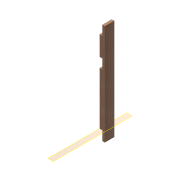
# Autodesk Inventor part: horizontalUnderSink
Saved by Autodesk Inventor 2018 (Build 220112000, 112)
## iProperties
Created: 2018-01-02
Part Number: horizontalUnderSink
Material: Wood (Birch)
Document SubType Name: Modeling
Designer: sawaiz
Density: 0.55 g/cm^3
Appearance: Birch - Natural Polished
Author: sawaiz
Autodesk Inventor part; units mm, degrees
ref_plane "Work Plane1" through (0, 0, 0) normal (0, 0, 1) x (1, 0, 0)
sketch "Sketch1" plane through (0, 0, 0) normal (0, 0, 1) x (1, 0, 0)
  line L0 (29, 140) -> (29, 248) projected
  line L1 (29, 248) -> (58, 248) projected
  line L2 (29, 248) -> (58, 248) projected
  line L3 (58, 248) -> (58, 410) projected
  line L4 (0, 410) -> (58, 410) projected
  line L5 (0, -410) -> (0, 410) projected
  line L6 (58, -410) -> (0, -410) projected
  line L7 (58, -410) -> (58, -252) projected
  line L8 (58, -252) -> (29, -252) projected
  line L9 (29, -252) -> (29, -144) projected
  line L10 (29, -144) -> (58, -144) projected
  line L11 (58, -144) -> (58, 140) projected
  line L12 (58, 140) -> (29, 140) projected
  line L13 (29, 140) -> (29, 248) projected
  line L14 (58, 140) -> (29, 140) projected
  line L15 (58, 140) -> (0, 140)
  line L16 (0, 140) -> (0, 248)
  line L17 (0, 248) -> (58, 248)
  line L18 (58, 248) -> (58, 140)
  point P0 (0, 0)
  constraints: 8 end point, 2 parallel, 1 horizontal, 1 perpendicular, 1 point on line
ref_plane "Work Plane2" through (0, -410, -108) normal (0, 0, -1) x (0, 1, 0)
ref_plane "Work Plane3" through (0, -410, 1041.034) normal (0, 0, 1) x (1, 0, 0)
extrude "Extrusion1" add sketch "Sketch1" along normal up to surface (1149.034 mm away) from surface at -108 contours L15 L5 L17 L0 | L0 L1 L18 L12
sketch "Sketch2" plane through (0, 140, 1041.034) normal (-1, 0, 0) x (0, 0, 1)
  line L0 (-1041.034, -550) -> (-1041.034, 270) projected
  line L1 (-1149.034, 270) -> (-1041.034, 270) projected
  line L2 (-1149.034, -550) -> (-1149.034, 270) projected
  line L3 (-1041.034, -550) -> (-1149.034, -550) projected
  line L4 (-333.034, -550) -> (-333.034, 270) projected
  line L5 (-441.034, 270) -> (-333.034, 270) projected
  line L6 (-441.034, -550) -> (-441.034, 270) projected
  line L7 (-333.034, -550) -> (-441.034, -550) projected
  line L8 (0, -550) -> (0, 270) projected
  line L9 (-108, 270) -> (0, 270) projected
  line L10 (-108, -550) -> (-108, 270) projected
  line L11 (0, -550) -> (-108, -550) projected
  line L12 (0, 0) -> (0, 108) projected
  line L13 (-1149.034, 108) -> (0, 108) projected
  line L14 (-1149.034, 108) -> (-1149.034, 0) projected
  line L15 (-1149.034, 0) -> (0, 0) projected
  line L16 (-1041.034, 0) -> (-1149.034, 0)
  line L17 (-1149.034, 0) -> (-1149.034, 108)
  line L18 (-1149.034, 108) -> (-1041.034, 108)
  line L19 (-1041.034, 108) -> (-1041.034, 0)
  line L20 (-1149.034, 108) -> (0, 108) projected
  line L21 (-441.034, 108) -> (-333.034, 108)
  line L22 (-333.034, 108) -> (-333.034, 0)
  line L23 (-333.034, 0) -> (-441.034, 0)
  line L24 (-441.034, 0) -> (-441.034, 108)
  line L25 (-1149.034, 0) -> (0, 0) projected
  line L26 (0, 0) -> (0, 108) projected
  line L27 (-108, 0) -> (0, 0)
  line L28 (0, 0) -> (0, 108)
  line L29 (0, 108) -> (-108, 108)
  line L30 (-108, 108) -> (-108, 0)
  point P0 (-1041.034, -140)
  constraints: 24 end point, 8 point on line, 6 parallel, 3 horizontal, 3 perpendicular
ref_plane "Work Plane4" through (29, 140, 933.034) normal (1, 0, 0) x (0, 1, 0)
extrude "Extrusion2" cut sketch "Sketch2" against normal up to surface (29 mm away) contours L15 L2 L13 L0 | L6 L13 L4 L15 | L10 L13 L8 L15
body "Solid1"
